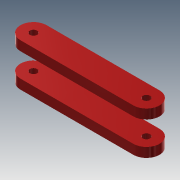
# Autodesk Inventor part: biela-dedo-2
Saved by Autodesk Inventor 2017 (Build 210142000, 142)
## iProperties
Created: 2018-05-30
Part Number: biela-dedo-2
Material: Generic
Document SubType Name: Modeling
Designer: Luiz Gustavo
Density: 1 g/cm^3
Appearance: Smooth - Red
Mass: 4.63032 g
Surface Area: 36.0371 cm^2
Volume: 4.63032 cm^3
Author: Luiz Gustavo
Autodesk Inventor part; units mm, degrees
ref_plane "YZ Plane" through (0, 0, 0) normal (1, 0, 0) x (0, 1, 0)
ref_plane "XZ Plane" through (0, 0, 0) normal (0, 1, 0) x (-1, 0, 0)
ref_plane "XY Plane" through (0, 0, 0) normal (0, 0, 1) x (1, 0, 0)
sketch "Sketch1" plane through (0, 0, 0) normal (0, 0, 1) x (1, 0, 0)
  line L0 (-50.2197, 25) -> (-2.6718, 25) construction
  circle A0 centre (-50.2197, 25) radius 1.55
  arc A1 (-50.2197, 19.5) -> (-50.2197, 30.5) centre (-50.2197, 25) ccw construction
  circle A2 centre (-2.6718, 25) radius 1.55
  arc A3 (-2.6718, 30.5) -> (-2.6718, 19.5) centre (-2.6718, 25) ccw construction
  line L1 (-50.2197, 30.5) -> (-2.6718, 30.5)
  line L2 (-50.2197, 19.5) -> (-2.6718, 19.5)
  arc A4 (-50.2197, 30.5) -> (-50.2197, 19.5) centre (-50.2197, 25) ccw
  arc A5 (-2.6718, 19.5) -> (-2.6718, 30.5) centre (-2.6718, 25) ccw
  point P0 (0, 0)
  dimension "d0" = 11
  dimension "d1" = 3.1
  constraints: 8 point on circle, 6 centre point, 4 coincident, 4 end point, 3 tangent, 2 equal radius, 1 horizontal
  measures "d0" diameter of A3
  measures "d1" diameter of A2
extrude "Extrusion1" add sketch "Sketch1" along normal mid plane 18
sketch "Sketch2" plane through (0, 0, 0) normal (0, 0, 1) x (1, 0, 0)
  circle A0 centre (-2.6718, 25) radius 1.55 projected
  circle A1 centre (-50.2197, 25) radius 1.55 projected
  line L0 (-2.6718, 30.5) -> (-50.2197, 30.5) projected
  arc A2 (-50.2197, 30.5) -> (-50.2197, 19.5) centre (-50.2197, 25) ccw projected
  line L1 (-50.2197, 19.5) -> (-2.6718, 19.5) projected
  arc A3 (-2.6718, 19.5) -> (-2.6718, 30.5) centre (-2.6718, 25) ccw projected
  point P0 (0, 0)
extrude "Extrusion2" cut sketch "Sketch2" along normal mid plane 10
body "Solid1"
